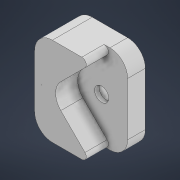
# Autodesk Inventor part: corner fitter
Saved by Autodesk Inventor 2022 (Build 260153000, 153)
## iProperties
Created: 2023-05-22
Part Number: corner fitter
Material: Generic
Document SubType Name: Modeling
Designer: Jakob Saugbjerg
Density: 1 g/cm^3
Appearance: Default
Author: Jakob Saugbjerg
Autodesk Inventor part; units mm, degrees
ref_plane "YZ Plane" through (0, 0, 0) normal (1, 0, 0) x (0, 1, 0)
ref_plane "XZ Plane" through (0, 0, 0) normal (0, 1, 0) x (-1, 0, 0)
ref_plane "XY Plane" through (0, 0, 0) normal (0, 0, 1) x (1, 0, 0)
sketch "Sketch1" plane through (0, 0, 0) normal (0, 0, 1) x (1, 0, 0)
  line L0 (0, 0) -> (20, 0)
  line L1 (20, 0) -> (20, 10)
  line L2 (20, 10) -> (0, 10)
  line L3 (0, 10) -> (0, 0)
  dimension "d0" = 20
  dimension "d1" = 10
  constraints: 8 end point, 2 parallel, 1 horizontal, 1 perpendicular
  measures "d0" distance of L2.end L1.end
  measures "d1" distance of L1.end L0.end
sketch "Sketch1 outline for Extrusion1" plane through (0, 0, 0) normal (0, 0, 1) x (1, 0, 0)
  line L0 (0, 0) -> (20, 0)
  line L1 (0, 10) -> (0, 0)
  line L2 (20, 10) -> (0, 10)
  line L3 (20, 0) -> (20, 10)
extrude "Extrusion1" add sketch "Sketch1 outline for Extrusion1" along normal blind 4
sketch "Sketch2" plane through (0, 0, 4) normal (0, 0, 1) x (1, 0, 0)
  line L0 (0, 10) -> (0, 0) projected
  line L1 (0, 5) -> (7.071, 5)
  line L2 (7.071, 5) -> (14.142, 5)
  circle A0 centre (7.071, 5) radius 1.6
  circle A1 centre (14.142, 5) radius 2.95
  dimension "d4" = 7.071
  dimension "d5" = 7.071
  dimension "d6" = 3.2
  dimension "d7" = 5.9
  constraints: 4 end point, 2 centre point, 2 coincident, 1 horizontal, 1 midpoint, 1 point on line
  measures "d4" distance of L1.start L1.end
  measures "d5" distance of L1.end L2.end
  measures "d6" diameter of A0
  measures "d7" diameter of A1
sketch "Sketch2 outline for Extrusion2" plane through (0, 0, 4) normal (0, 0, 1) x (1, 0, 0)
  circle A0 centre (7.071, 5) radius 1.6
extrude "Extrusion2" cut sketch "Sketch2 outline for Extrusion2" against normal blind 4
sketch "Sketch3" plane through (0, 0, 4) normal (0, 0, 1) x (1, 0, 0)
  circle A0 centre (7.071, 5) radius 1.6 projected
  line L0 (7.071, 5) -> (14.142, 5)
  circle A1 centre (14.142, 5) radius 1.6
  point P0 (0, 0)
  dimension "d10" = 7.071
  dimension "d11" = 3.2
  constraints: 2 end point, 1 centre point, 1 coincident, 1 horizontal
  measures "d10" distance of L0.start L0.end
  measures "d11" diameter of A1
sketch "Sketch3 outline for Extrusion3" plane through (0, 0, 4) normal (0, 0, 1) x (1, 0, 0)
  circle A0 centre (14.142, 5) radius 1.6
extrude "Extrusion3" cut sketch "Sketch3 outline for Extrusion3" against normal blind 3
sketch "Sketch5" plane through (0, 0, 4) normal (0, 0, 1) x (1, 0, 0)
  line L0 (0, 0) -> (20, 0) projected
  line L1 (0, 10) -> (4, 10)
  line L2 (4, 10) -> (4, 0)
  line L3 (4, 0) -> (0, 0)
  line L4 (0, 0) -> (0, 10)
  dimension "d17" = 4
  constraints: 8 end point, 2 parallel, 1 horizontal, 1 perpendicular, 1 point on line
  measures "d17" distance of L2.end L3.end
sketch "Sketch5 outline for Extrusion5" plane through (0, 0, 4) normal (0, 0, 1) x (1, 0, 0)
  line L0 (4, 10) -> (0, 10)
  line L1 (4, 0) -> (4, 10)
  line L2 (0, 0) -> (4, 0)
  line L3 (0, 10) -> (0, 0)
extrude "Extrusion5" cut sketch "Sketch5 outline for Extrusion5" against normal blind 4
sketch "Sketch6" plane through (0, 0, 4) normal (0, 0, 1) x (1, 0, 0)
  circle A0 centre (7.071, 5) radius 1.6
  line L0 (7.071, 5) -> (9.899427, 7.828427)
  line L1 (7.071, 5) -> (11.071, 5) construction
  line L2 (20, 10) -> (4, 10)
  line L3 (4, 0) -> (20, 0)
  line L4 (7.071, 5) -> (5.414, 5)
  line L5 (5.414, 5) -> (8.242427, 7.828427)
  line L6 (5.414, 5) -> (9.414, 5) construction
  line L7 (5.414, 5) -> (10.414, 0)
  line L8 (5.414, 5) -> (12.485068, 5) construction
  arc A1 (8.242427, 7.828427) -> (8.242427, 2.171573) centre (11.070854, 5) ccw
  circle A2 centre (7.071, 5) radius 1.6
  line L9 (20, 10) -> (4, 10)
  arc A3 (8.914, 10) -> (10.414, 0) centre (9.664, 5) ccw
  line L10 (8.914, 10) -> (4, 10)
  line L11 (4, 10) -> (4, 0)
  line L12 (4, 0) -> (8.914, 0)
  line L13 (8.914, 0) -> (8.914, 10)
  line L14 (7.071, 5) -> (12.071, 0)
  line L15 (4, 0) -> (20, 0)
  line L16 (7.071, 5) -> (14.142068, 5) construction
  line L17 (9.899427, 7.828427) -> (12.071, 10)
  arc A4 (9.899427, 7.828427) -> (9.899427, 2.171573) centre (12.727854, 5) ccw
  line L18 (8.242427, 7.828427) -> (10.414, 10)
  point P0 (0, 0)
  point P1 (13.001674, 10)
  point P2 (10.571, 0)
  point P3 (9.364849, 1.723072)
  point P4 (8.914, 10)
  point P5 (8.914, 0)
  point P6 (7.390866, 3.432299)
  point P7 (5.472054, 4.941946)
  point P8 (5.472054, 5.058054)
  point P9 (7.390866, 6.567701)
  point P10 (7.012946, 3.401054)
  point P11 (8.914, 1.5)
  point P12 (8.914, 0)
  point P13 (8.914, 10)
  point P14 (8.914, 8.5)
  dimension "d21" = 4
  dimension "d22" = 45
  dimension "d24" = 1.657
  dimension "d25" = 45
  dimension "d26" = 45
  dimension "d27" = 4
  dimension "d35" = 45
  dimension "d36" = 4
  constraints: 30 end point, 10 point on line, 6 point on circle, 5 horizontal, 4 centre point, 4 equal length, 2 parallel, 1 coincident, 1 perpendicular, 1 tangent
  measures "d21" distance of L0.start L0.end
  measures "d22" angle of L1 L0
  measures "d24" distance of L0.start L4.end
  measures "d25" angle of L6 L5
  measures "d26" angle of L7 L8
  measures "d27" radius of A1
  measures "d35" angle of L14 L16
  measures "d36" radius of A4
sketch "Sketch6 outline for Extrusion6" plane through (0, 0, 4) normal (0, 0, 1) x (1, 0, 0)
  line L0 (5.472054, 4.941946) -> (5.414, 5)
  line L1 (5.414, 5) -> (5.472054, 5.058054)
  arc A0 (5.472054, 5.058054) -> (5.472054, 4.941946) centre (7.071, 5) cw
  line L2 (12.071, 10) -> (4, 10)
  line L3 (4, 10) -> (4, 0)
  line L4 (4, 0) -> (12.071, 0)
  line L5 (12.071, 0) -> (9.899427, 2.171573)
  arc A1 (9.899427, 2.171573) -> (9.899427, 7.828427) centre (12.727854, 5) cw
  line L6 (9.899427, 7.828427) -> (12.071, 10)
extrude "Extrusion6" add sketch "Sketch6 outline for Extrusion6" along normal blind 5
sketch "Sketch8" plane through (0, 0, 0) normal (0, 0, -1) x (-1, 0, 0)
  circle A0 centre (-14.142, 5) radius 1.6 projected
  circle A1 centre (-14.142, 5) radius 2.95
  point P0 (0, 0)
  dimension "d37" = 5.9
  constraints: 1 centre point, 1 coincident
  measures "d37" diameter of A1
sketch "Sketch8 outline for Extrusion8" plane through (0, 0, 0) normal (0, 0, -1) x (-1, 0, 0)
  circle A0 centre (-14.142, 5) radius 2.95
extrude "Extrusion8" cut sketch "Sketch8 outline for Extrusion8" against normal blind 3
sketch "Sketch9" plane through (0, 0, 0) normal (0, 0, -1) x (-1, 0, 0)
  arc A0 (-5.472054, 5.058054) -> (-5.472054, 4.941946) centre (-7.071, 5) ccw
  circle A1 centre (-7.071, 5) radius 2.95
  point P0 (0, 0)
  dimension "d40" = 5.9
  constraints: 1 centre point, 1 coincident
  measures "d40" diameter of A1
sketch "Sketch9 outline for Extrusion9" plane through (0, 0, 0) normal (0, 0, -1) x (-1, 0, 0)
  circle A0 centre (-7.071, 5) radius 2.95
extrude "Extrusion9" cut sketch "Sketch9 outline for Extrusion9" against normal blind 3.9
sketch "Sketch10" plane through (0, 0, 9) normal (0, 0, 1) x (1, 0, 0)
  arc A0 (5.472054, 4.941946) -> (5.472054, 5.058054) centre (7.071, 5) ccw
  circle A1 centre (7.071, 5) radius 1.6
  point P0 (0, 0)
  point P1 (5.472054, 5.058054)
  constraints: 1 coincident, 3 other
sketch "Sketch10 outline for Extrusion10" plane through (0, 0, 9) normal (0, 0, 1) x (1, 0, 0)
  arc A0 (5.472054, 5.058054) -> (5.472054, 4.941946) centre (7.071, 5) ccw
  arc A1 (5.472054, 4.941946) -> (5.472054, 5.058054) centre (7.071, 5) ccw
extrude "Extrusion10" add sketch "Sketch10 outline for Extrusion10" against normal blind 5.1
sketch "Sketch11" plane through (12.071, 10, 9) normal (0, 1, 0) x (1, 0, 0)
  line L0 (-8.071, 0) -> (-8.071, 9) projected
  line L1 (7.929, 9) -> (7.929, 5) projected
  line L2 (-8.071, 9) -> (7.929, 9)
  line L3 (7.929, 9) -> (7.929, 5)
  line L4 (7.929, 5) -> (-8.071, 5)
  line L5 (-8.071, 5) -> (-8.071, 9)
  point P0 (-12.071, 9)
  constraints: 8 end point, 2 parallel, 1 horizontal, 1 perpendicular
sketch "Sketch11 outline for Extrusion11" plane through (12.071, 10, 9) normal (0, 1, 0) x (1, 0, 0)
  line L0 (7.929, 9) -> (-8.071, 9)
  line L1 (7.929, 5) -> (7.929, 9)
  line L2 (-8.071, 5) -> (7.929, 5)
  line L3 (-8.071, 9) -> (-8.071, 5)
extrude "Extrusion11" add sketch "Sketch11 outline for Extrusion11" along normal blind 5
sketch "Sketch12" plane through (20, 0, 0) normal (0, -1, 0) x (1, 0, 0)
  line L0 (0, 4) -> (0, 0) projected
  line L1 (-7.929, 4) -> (-16, 4) projected
  line L2 (0, 0) -> (-16, 0)
  line L3 (-16, 0) -> (-16, 4)
  line L4 (-16, 4) -> (0, 4)
  line L5 (0, 4) -> (0, 0)
  point P0 (-20, 0)
  constraints: 8 end point, 2 parallel, 1 horizontal, 1 perpendicular
sketch "Sketch12 outline for Extrusion12" plane through (20, 0, 0) normal (0, -1, 0) x (1, 0, 0)
  line L0 (-16, 4) -> (-16, 0)
  line L1 (-7.929, 4) -> (-16, 4)
  line L2 (0, 4) -> (-7.929, 4)
  line L3 (0, 0) -> (0, 4)
  line L4 (-16, 0) -> (0, 0)
extrude "Extrusion12" add sketch "Sketch12 outline for Extrusion12" along normal blind 5
sketch "Sketch13" plane through (0, 0, 4) normal (0, 0, 1) x (1, 0, 0)
  line L0 (9.899427, 2.171573) -> (12.071, 0)
  line L1 (12.071, 10) -> (9.899427, 7.828427)
  line L2 (12.071, 10) -> (17.071, 15)
  line L3 (20, 15) -> (4, 15)
  line L4 (12.071, 10) -> (19.142068, 10) construction
  line L5 (20, 15) -> (20, -5)
  line L6 (12.071, 10) -> (4, 10)
  line L7 (4, 10) -> (17.071, 10)
  line L8 (17.071, 10) -> (17.071, 15)
  line L9 (17.071, 15) -> (4, 15)
  line L10 (4, 15) -> (4, 10)
  line L11 (12.071, 0) -> (17.071, -5)
  line L12 (12.071, 0) -> (19.142068, 0) construction
  line L13 (4, 0) -> (12.071, 0)
  line L14 (4, 0) -> (20, 0)
  line L15 (20, 0) -> (20, -5)
  line L16 (20, -5) -> (4, -5)
  line L17 (4, -5) -> (4, 0)
  dimension "d50" = 45
  dimension "d51" = 45
  constraints: 24 end point, 4 horizontal, 4 parallel, 2 equal length, 2 perpendicular, 1 point on line
  measures "d50" angle of L4 L2
  measures "d51" angle of L11 L12
sketch "Sketch13 outline for Extrusion13" plane through (0, 0, 4) normal (0, 0, 1) x (1, 0, 0)
  line L0 (4, 15) -> (4, 10)
  line L1 (17.071, 15) -> (4, 15)
  line L2 (12.071, 10) -> (17.071, 15)
  line L3 (4, 10) -> (12.071, 10)
  line L4 (4, 0) -> (4, -5)
  line L5 (12.071, 0) -> (4, 0)
  line L6 (17.071, -5) -> (12.071, 0)
  line L7 (4, -5) -> (17.071, -5)
extrude "Extrusion13" add sketch "Sketch13 outline for Extrusion13" along normal blind 5
fillet "Fillet2" radius 4 4 edges at (20, 15, 2) (4, 15, 4.5) (20, -5, 2) (4, -5, 4.5)
fillet "Fillet3" radius 1 2 edges at (16.9553, 14.8843, 6.5) (16.9553, -4.8843, 6.5)
body "Solid1"
